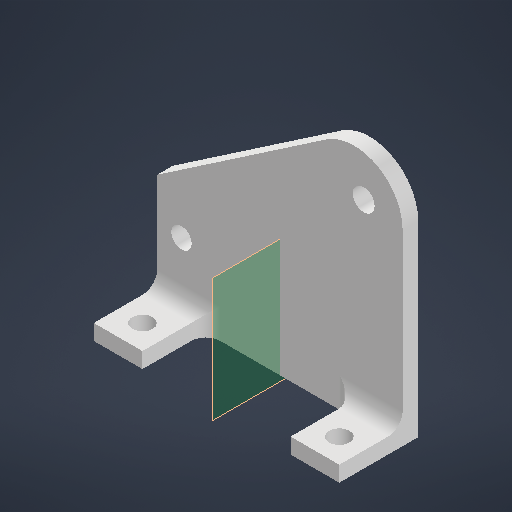
# Autodesk Inventor part: мертвое колесо 3
Saved by Autodesk Inventor 2026.2 (Build 302298000, 298)
## iProperties
Created: 2025-09-25
Part Number: мертвое колесо 3
Material: Типовые
Document SubType Name: Modeling
Designer: GameHD
Density: 1 g/cm^3
Appearance: По умолчанию
Author: GameHD
Autodesk Inventor part; units mm, degrees
ref_plane "YZ Plane" through (0, 0, 0) normal (1, 0, 0) x (0, 1, 0)
ref_plane "XZ Plane" through (0, 0, 0) normal (0, 1, 0) x (-1, 0, 0)
ref_plane "XY Plane" through (0, 0, 0) normal (0, 0, 1) x (1, 0, 0)
sketch "Эскиз1" plane through (0, 0, 0) normal (0, 0, 1) x (1, 0, 0)
  circle A0 centre (0, 0) radius 2.1
  line L0 (-5, 14.35) -> (5, 14.35)
  line L1 (5, 14.35) -> (5, -14.35)
  line L2 (5, -14.35) -> (-5, -14.35)
  line L3 (-5, -14.35) -> (-5, 14.35)
  line L4 (-5, 14.35) -> (5, -14.35) construction
  line L5 (5, 14.35) -> (-5, -14.35) construction
  line L6 (-5, 7) -> (5, 7)
  dimension "d0" = 4.2
  dimension "d2" = 10
  dimension "d3" = 28.7
  dimension "d4" = 7
  constraints: 14 end point, 2 midpoint, 2 parallel, 2 perpendicular, 2 point on line, 1 centre point, 1 coincident, 1 horizontal
  measures "d0" diameter of A0
  measures "d2" distance of L1.end L2.end
  measures "d3" distance of L2.end L0.start
  measures "d4" distance from line of A0.centre L6
extrude "Выдавливание1" add sketch "Эскиз1" along normal blind 3.2 contours L6 L1 L2 L3
sketch "Эскиз2" plane through (0, 0, 3.2) normal (0, 0, 1) x (1, 0, 0)
  line L0 (5, -14.35) -> (5, 7) projected
  line L1 (5, -14.35) -> (-5, -14.35)
  line L2 (-5, -14.35) -> (-5, -11.15)
  line L3 (-5, -11.15) -> (5, -11.15)
  line L4 (5, -11.15) -> (5, -14.35)
  point P0 (0, 0)
  point P1 (5, -11.15)
  dimension "d7" = 10
  dimension "d8" = 3.2
  constraints: 8 end point, 2 parallel, 1 horizontal, 1 perpendicular
  measures "d7" distance of L2.end L3.end
  measures "d8" distance of L1.end L2.end
extrude "Выдавливание2" add sketch "Эскиз2" along normal blind 13
fillet "Сопряжение1" radius 3 1 edges at (0, -11.15, 3.2)
sketch "Эскиз3" plane through (-5, -11.15, 16.2) normal (0, 1, 0) x (1, 0, 0)
  line L0 (0, 10) -> (10, 10) projected
  line L1 (5, 10) -> (5, 0)
  line L2 (0, 0) -> (10, 0) projected
  circle A0 centre (5, 5) radius 2.1
  point P0 (5, 16.2)
  dimension "d12" = 4.2
  constraints: 3 midpoint, 2 end point, 1 centre point
  measures "d12" diameter of A0
extrude "Выдавливание3" cut sketch "Эскиз3" against normal blind 13
sketch "Эскиз4" plane through (0, 0, 3.2) normal (0, 0, 1) x (1, 0, 0)
  circle A0 centre (37.4046, 25.4735) radius 2.6917 projected
  line L0 (35.1798, 23.9584) -> (0, 0)
  line L1 (29.7757, 32.3768) -> (-5, 8.6936)
  line L2 (-5, 7) -> (-5, -8.15) projected
  line L3 (-5, 7) -> (-5, 8.6936)
  line L4 (-5, -14.35) -> (5, -14.35) projected
  line L5 (5, -14.35) -> (5, -11.15) projected
  line L6 (5, -11.15) -> (-5, -11.15) projected
  line L7 (-5, -11.15) -> (-5, -14.35) projected
  line L8 (37.4046, 25.4735) -> (37.4046, -14.35)
  line L9 (45.4046, 24.1114) -> (45.4046, -14.35)
  arc A1 (45.4046, 24.1114) -> (29.7757, 32.3768) centre (35.4046, 24.1114) ccw
  line L10 (-5, -14.35) -> (45.4046, -14.35)
  circle A2 centre (37.4046, 25.4735) radius 2.25
  line L11 (-5, 8.6936) -> (-5, -14.35)
  circle A3 centre (0, 0) radius 2.1 projected
  dimension "d15" = 10
  dimension "d16" = 8
  dimension "d17" = 10
  dimension "d18" = 4.5
  constraints: 14 end point, 2 centre point, 2 parallel, 2 point on circle, 2 tangent, 2 vertical, 1 coincident, 1 horizontal, 1 perpendicular, 2 other
  measures "d15" distance from line of L8.start L1
  measures "d16" distance between parallel lines of L8 L9
  measures "d17" radius of A1
  measures "d18" diameter of A2
extrude "Выдавливание4" add sketch "Эскиз4" against normal up to surface (3.2 mm away) contours A0 | A1 L9 L10 L5 L6 L11 L2 L3 L1
fillet "Сопряжение2" radius 3 1 edges at (5, -11.25, 3.2)
ref_plane "РабПлоскость1" through (20.202, -14.35, 16.2) normal (-1, 0, 0) x (0, 0, 1)
mirror "Зеркальное отражение1" about plane through (20.202, -14.35, 16.2) normal (-1, 0, 0) of "Выдавливание2", "Выдавливание3", "Сопряжение1", "Сопряжение2"
